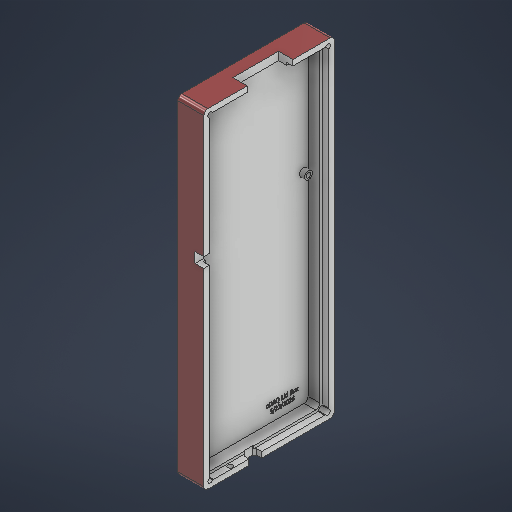
# Autodesk Inventor part: cDAQ_Lid_Box
Saved by Autodesk Inventor 2027 (Build 310192000, 192)
## iProperties
Created: 2026-05-08
Part Number: cDAQ_Lid_Box
Material: Generic
Document SubType Name: Modeling
Designer: giese
Density: 1 g/cm^3
Appearance: Default
Author: giese
Autodesk Inventor part; units mm, degrees
(part 1 of 2)
ref_plane "YZ Plane" through (0, 0, 0) normal (1, 0, 0) x (0, 1, 0)
ref_plane "XZ Plane" through (0, 0, 0) normal (0, 1, 0) x (-1, 0, 0)
ref_plane "XY Plane" through (0, 0, 0) normal (0, 0, 1) x (1, 0, 0)
sketch "Sketch1" plane through (0, 0, 0) normal (1, 0, 0) x (0, 1, 0)
  line L0 (50.7569, 48.4212) -> (-205.7831, 48.4212)
  line L1 (-205.7831, 48.4212) -> (-205.7831, -53.1788)
  line L2 (-205.7831, -53.1788) -> (50.7569, -53.1788)
  line L3 (50.7569, -53.1788) -> (50.7569, 48.4212)
  point P0 (0, 0)
  dimension "d0" = 101.6
  dimension "d1" = 256.54
  constraints: 8 end point, 2 parallel, 1 horizontal, 1 perpendicular
  measures "d0" distance of L2.end L0.start
  measures "d1" distance of L0.start L0.end
extrude "Extrusion1" add sketch "Sketch1" along normal blind 20.32
sketch "Sketch2" plane through (20.32, 0, 0) normal (1, 0, 0) x (0, 0, -1)
  line L0 (-42.0712, 44.4069) -> (46.8288, 44.4069)
  line L1 (46.8288, 44.4069) -> (46.8288, -199.4331)
  line L2 (46.8288, -199.4331) -> (-42.0712, -199.4331)
  line L3 (-42.0712, -199.4331) -> (-42.0712, 44.4069)
  line L4 (-48.4212, 50.7569) -> (-48.4212, -205.7831) projected
  line L5 (-48.4212, -205.7831) -> (53.1788, -205.7831) projected
  point P0 (0, 0)
  dimension "d4" = 88.9
  dimension "d5" = 243.84
  dimension "d6" = 6.35
  dimension "d7" = 6.35
  constraints: 8 end point, 2 parallel, 1 horizontal, 1 perpendicular
  measures "d4" distance of L0.start L0.end
  measures "d5" distance of L0.end L1.end
  measures "d6" distance between parallel lines of L4 L3
  measures "d7" distance between parallel lines of L5 L2
extrude "Extrusion2" cut sketch "Sketch2" against normal blind 13.97
sketch "Sketch3" plane through (0, 0, 0) normal (-1, 0, 0) x (0, 0, 1)
  circle A0 centre (-30.3188, 7.3229) radius 2
  line L0 (-53.1788, -205.7831) -> (-53.1788, 50.7569) projected
  line L1 (-53.1788, 50.7569) -> (48.4212, 50.7569) projected
  circle A1 centre (-11.82, 7.3229) radius 2
  circle A2 centre (6.6789, 7.3229) radius 2
  point P0 (0, 0)
  dimension "d10" = 22.86
  dimension "d11" = 43.434
  dimension "d12" = 43.434
  dimension "d13" = 18.4988
  dimension "d14" = 4
  dimension "d15" = 4
  dimension "d16" = 43.434
  dimension "d17" = 18.4988
  dimension "d18" = 36.9976
  dimension "d21" = 4
  constraints: 3 centre point
  measures "d10" distance from line of L0 A0.centre
  measures "d11" distance from line of L1 A0.centre
  measures "d12" distance from line of L1 A1.centre
  measures "d13" distance of A0.centre A1.centre
  measures "d14" diameter of A1
  measures "d15" diameter of A2
  measures "d16" distance from line of L1 A2.centre
  measures "d17" distance of A1.centre A2.centre
  measures "d18" distance of A0.centre A2.centre
  measures "d21" diameter of A0
extrude "Extrusion3" [suppressed]
sketch "Sketch6" plane through (0, 50.7569, 48.4212) normal (0, 1, 0) x (1, 0, 0)
  line L0 (20.32, 6.35) -> (20.32, 95.25) projected
  line L1 (9.144, 33.7719) -> (20.32, 33.7719)
  line L2 (20.32, 33.7719) -> (20.32, 69.342)
  line L3 (20.32, 69.342) -> (9.144, 69.342)
  line L4 (9.144, 69.342) -> (9.144, 33.7719)
  line L5 (0, 101.6) -> (20.32, 101.6) projected
  point P0 (0, 48.4212)
  point P1 (14.732, 69.342)
  point P2 (14.732, 33.7719)
  dimension "d30" = 11.176
  dimension "d31" = 35.5701
  dimension "d32" = 32.258
  constraints: 8 end point, 2 midpoint, 2 parallel, 1 horizontal, 1 perpendicular, 1 point on line
  measures "d30" distance between parallel lines of L0 L4
  measures "d31" distance of point (14.732, 69.342) point (14.732, 33.772)
  measures "d32" distance between parallel lines of L5 L3
extrude "Extrusion5" cut sketch "Sketch6" against normal blind 6.35
fillet "Fillet1" radius 3.175 4 edges at (10.16, 50.7569, -53.1788) (10.16, 50.7569, 48.4212) (10.16, -205.7831, 48.4212) (10.16, -205.7831, -53.1788)
sketch "Sketch7" plane through (20.32, 0, 0) normal (1, 0, 0) x (0, 0, -1)
  line L0 (-42.0712, -199.4331) -> (-42.0712, 44.4069) projected
  line L1 (-42.0712, 44.4069) -> (-42.3252, 44.4069)
  line L2 (-42.3252, 46.4069) -> (-44.0712, 46.4069)
  line L3 (-44.0712, 46.4069) -> (-44.0712, 51.0109)
  line L4 (-42.0712, -190.1621) -> (-42.0712, -199.4331)
  line L5 (46.8288, -199.4331) -> (-42.0712, -199.4331) projected
  line L6 (-40.4202, -201.4331) -> (-44.0712, -201.4331)
  line L7 (-44.0712, -201.4331) -> (-44.0712, -190.1621)
  line L8 (46.8288, 44.4069) -> (46.8288, -199.4331) projected
  line L9 (46.8288, -192.7021) -> (46.8288, -199.4331)
  line L10 (46.8288, -199.4331) -> (43.9078, -199.4331)
  line L11 (46.8288, -199.4331) -> (46.8288, -192.7021)
  line L12 (48.8288, -192.7021) -> (48.8288, -201.4331)
  line L13 (48.8288, -201.4331) -> (43.9078, -201.4331)
  line L14 (-42.0712, 44.4069) -> (46.8288, 44.4069) projected
  line L15 (42.0028, 44.4069) -> (46.8288, 44.4069)
  line L16 (48.8288, 48.4709) -> (48.8288, 46.4069)
  line L17 (48.8288, 46.4069) -> (42.0028, 46.4069)
  line L18 (-42.3252, 46.4069) -> (42.0028, 46.4069)
  line L19 (42.0028, 44.4069) -> (-42.3252, 44.4069)
  line L20 (48.8288, 48.4709) -> (48.8288, -192.7021)
  line L21 (44.2888, -195.2421) -> (44.2888, 44.4069)
  line L22 (43.9078, -199.4331) -> (-40.4202, -199.4331)
  line L23 (-40.4202, -201.4331) -> (43.9078, -201.4331)
  line L24 (-44.0712, -190.1621) -> (-44.0712, 51.0109)
  line L25 (-42.0712, 44.4069) -> (-42.0712, -190.1621)
  point P0 (0, 0)
  point P1 (-42.0712, 51.0109)
  point P2 (-44.2302, 48.9789)
  point P3 (46.8288, 48.4709)
  point P4 (48.8288, 46.4069)
  dimension "d34" = 2
  dimension "d35" = 2
  dimension "d38" = 2
  dimension "d39" = 2
  dimension "d42" = 2
  dimension "d43" = 2
  dimension "d46" = 2
  dimension "d47" = 2
  constraints: 44 end point, 9 point on line, 4 parallel, 4 perpendicular, 2 collinear, 2 horizontal, 2 vertical
  measures "d34" distance between parallel lines of L2 L1
  measures "d35" distance between parallel lines of L0 L3
  measures "d38" distance between parallel lines of L7 L0
  measures "d39" distance between parallel lines of L5 L6
  measures "d42" distance between parallel lines of L5 L13
  measures "d43" distance between parallel lines of L8 L12
  measures "d46" distance between parallel lines of L14 L17
  measures "d47" distance between parallel lines of L8 L16
extrude "Extrusion6" cut sketch "Sketch7" against normal blind 5 contours L0 L14 L8 L5 | L18 L17 L20 L12 L13 L23 L6 L7 L24 L2
fillet "Fillet2" radius 3.175 6 edges at (10.835, 44.4069, 42.0712) (10.835, 44.4069, -46.8288) (10.835, -199.4331, 42.0712) (17.82, -201.4331, 44.0712) (10.835, -199.4331, -46.8288) (17.82, -201.4331, -48.8288)
sketch "Sketch11" plane through (15.32, 0, 0) normal (1, 0, 0) x (0, 0, -1)
  circle A0 centre (48.0988, 45.6769) radius 1.9939
  line L0 (50.0038, 50.7569) -> (20.9208, 50.7569) projected
  line L1 (53.1788, -202.6081) -> (53.1788, 47.5819) projected
  arc A1 (46.9238, 45.7719) -> (43.7488, 48.9469) centre (43.7488, 45.7719) ccw projected
  circle A2 centre (-43.3412, 45.6769) radius 1.9939
  line L2 (-48.4212, 47.5819) -> (-48.4212, -202.6081) projected
  line L3 (-14.6493, 50.7569) -> (-45.2462, 50.7569) projected
  circle A3 centre (48.0988, -200.7031) radius 1.9939
  line L4 (-45.2462, -205.7831) -> (50.0038, -205.7831) projected
  circle A4 centre (-43.3412, -200.7031) radius 1.9939
  circle A5 centre (43.0188, -43.2231) radius 1.9939
  circle A6 centre (-38.2612, -43.2231) radius 1.9939
  point P0 (0, 0)
  point P1 (45.9939, 48.017)
  point P2 (48.5528, -43.2993)
  point P3 (45.3778, -46.4743)
  point P4 (-30.4007, -42.8803)
  point P5 (-33.5757, -46.0553)
  dimension "d58" = 3.9878
  dimension "d59" = 5.08
  dimension "d60" = 5.08
  dimension "d61" = 3.9878
  dimension "d62" = 3.9878
  dimension "d63" = 5.08
  dimension "d64" = 5.08
  dimension "d65" = 3.9878
  dimension "d66" = 5.08
  dimension "d67" = 5.08
  dimension "d76" = 5.08
  dimension "d77" = 5.08
  dimension "d114" = 3.9878
  dimension "d115" = 93.98
  dimension "d116" = 10.16
  dimension "d117" = 3.9878
  dimension "d118" = 93.98
  dimension "d119" = 10.16
  constraints: 6 centre point, 1 point on circle
  measures "d58" diameter of A0
  measures "d59" distance from line of L2 A2.centre
  measures "d60" distance from line of L3 A2.centre
  measures "d61" diameter of A2
  measures "d62" diameter of A3
  measures "d63" distance from line of L1 A3.centre
  measures "d64" distance from line of L4 A3.centre
  measures "d65" diameter of A4
  measures "d66" distance from line of L2 A4.centre
  measures "d67" distance from line of L4 A4.centre
  measures "d76" distance from line of L1 A0.centre
  measures "d77" distance from line of L0 A0.centre
  measures "d114" diameter of A5
  measures "d115" distance from line of A5.centre L0
  measures "d116" distance from line of L1 A5.centre
  measures "d117" diameter of A6
  measures "d118" distance from line of A6.centre L3
  measures "d119" distance from line of L2 A6.centre
extrude "Extrusion8" cut sketch "Sketch11" along normal blind 5.08 and the other way blind 17.78
sketch "Sketch13" plane through (6.35, 0, 0) normal (1, 0, 0) x (0, 0, -1)
  line L0 (14.1785, -185.2739) -> (39.2344, -185.2739) construction
  line L1 (39.2344, -185.2739) -> (39.2344, -194.1382) construction
  line L2 (39.2344, -194.1382) -> (14.1785, -194.1382) construction
  line L3 (14.1785, -194.1382) -> (14.1785, -185.2739) construction
  spline S0 degree 2 poles (15.3666, -188.5097) (15.1295, -188.5097) (14.7367, -188.3639) (14.5959, -188.2157) knots 0 0 0 1 2 2 2
  spline S1 degree 2 poles (14.5959, -188.2157) (14.4552, -188.07) (14.2995, -187.6205) (14.2995, -187.3191) knots 0 0 0 1 2 2 2
  spline S2 degree 2 poles (14.2995, -187.3191) (14.2995, -187.0178) (14.4601, -186.5781) (14.5959, -186.4299) knots 0 0 0 1 2 2 2
  spline S3 degree 2 poles (14.5959, -186.4299) (14.7318, -186.2792) (15.1344, -186.1187) (15.3666, -186.1187) knots 0 0 0 1 2 2 2
  spline S4 degree 2 poles (15.3666, -186.1187) (15.5543, -186.1187) (15.9051, -186.2249) (16.0409, -186.2941) knots 0 0 0 1 2 2 2
  line L4 (16.0409, -186.2941) -> (16.0409, -186.7263)
  line L5 (16.0409, -186.7263) -> (16.0187, -186.7263)
  spline S5 degree 2 poles (16.0187, -186.7263) (15.9767, -186.6917) (15.8482, -186.6028) (15.7569, -186.5559) knots 0 0 0 1 2 2 2
  spline S6 degree 2 poles (15.7569, -186.5559) (15.6753, -186.5164) (15.458, -186.4546) (15.3592, -186.4546) knots 0 0 0 1 2 2 2
  spline S7 degree 2 poles (15.3592, -186.4546) (15.0603, -186.4546) (14.6972, -186.9066) (14.6972, -187.3191) knots 0 0 0 1 2 2 2
  spline S8 degree 2 poles (14.6972, -187.3191) (14.6972, -187.7217) (15.048, -188.1737) (15.3592, -188.1737) knots 0 0 0 1 2 2 2
  spline S9 degree 2 poles (15.3592, -188.1737) (15.5469, -188.1737) (15.8878, -188.0181) (16.0187, -187.8971) knots 0 0 0 1 2 2 2
  line L6 (16.0187, -187.8971) -> (16.0409, -187.8971)
  line L7 (16.0409, -187.8971) -> (16.0409, -188.3293)
  spline S10 degree 2 poles (16.0409, -188.3293) (15.9841, -188.3565) (15.8112, -188.4331) (15.742, -188.4504) knots 0 0 0 1 2 2 2
  spline S11 degree 2 poles (15.742, -188.4504) (15.6432, -188.48) (15.4876, -188.5097) (15.3666, -188.5097) knots 0 0 0 1 2 2 2
  spline S12 degree 2 poles (18.8246, -186.9363) (18.8246, -187.3537) (18.4862, -188.0255) (18.2022, -188.2133) knots 0 0 0 1 2 2 2
  spline S13 degree 2 poles (18.2022, -188.2133) (17.97, -188.359) (17.4933, -188.4578) (17.1228, -188.4578) knots 0 0 0 1 2 2 2
  line L8 (17.1228, -188.4578) -> (16.4213, -188.4578)
  line L9 (16.4213, -188.4578) -> (16.4213, -185.4098)
  line L10 (16.4213, -185.4098) -> (17.1154, -185.4098)
  spline S14 degree 2 poles (17.1154, -185.4098) (17.5451, -185.4098) (18.0342, -185.5382) (18.2071, -185.6519) knots 0 0 0 1 2 2 2
  spline S15 degree 2 poles (18.2071, -185.6519) (18.501, -185.847) (18.8246, -186.4917) (18.8246, -186.9363) knots 0 0 0 1 2 2 2
  spline S16 degree 2 poles (18.4022, -186.9313) (18.4022, -186.5806) (18.1701, -186.0841) (17.9404, -185.9433) knots 0 0 0 1 2 2 2
  spline S17 degree 2 poles (17.9404, -185.9433) (17.7773, -185.847) (17.4093, -185.7605) (17.1351, -185.7605) knots 0 0 0 1 2 2 2
  line L11 (17.1351, -185.7605) -> (16.8264, -185.7605)
  line L12 (16.8264, -185.7605) -> (16.8264, -188.107)
  line L13 (16.8264, -188.107) -> (17.1351, -188.107)
  spline S18 degree 2 poles (17.1351, -188.107) (17.4044, -188.107) (17.8119, -188.0206) (17.9774, -187.9045) knots 0 0 0 1 2 2 2
  spline S19 degree 2 poles (17.9774, -187.9045) (18.1898, -187.7612) (18.4022, -187.287) (18.4022, -186.9313) knots 0 0 0 1 2 2 2
  line L14 (18.9358, -188.4578) -> (19.9633, -185.4098)
  line L15 (19.9633, -185.4098) -> (20.4622, -185.4098)
  line L16 (20.4622, -185.4098) -> (21.4898, -188.4578)
  line L17 (21.4898, -188.4578) -> (21.0625, -188.4578)
  line L18 (21.0625, -188.4578) -> (20.7858, -187.6056)
  line L19 (20.7858, -187.6056) -> (19.6224, -187.6056)
  line L20 (19.6224, -187.6056) -> (19.3458, -188.4578)
  line L21 (19.3458, -188.4578) -> (18.9358, -188.4578)
  line L22 (20.6747, -187.2598) -> (20.2029, -185.8248)
  line L23 (20.2029, -185.8248) -> (19.7336, -187.2598)
  line L24 (19.7336, -187.2598) -> (20.6747, -187.2598)
  spline S20 degree 2 poles (24.3105, -189.2037) (24.1994, -189.2309) (23.9573, -189.2605) (23.8363, -189.2605) knots 0 0 0 1 2 2 2
  spline S21 degree 2 poles (23.8363, -189.2605) (23.4929, -189.2605) (23.0656, -188.8777) (23.0459, -188.522) knots 0 0 0 1 2 2 2
  spline S22 degree 2 poles (23.0459, -188.522) (23.0187, -188.522) (22.9718, -188.522) (22.952, -188.522) knots 0 0 0 1 2 2 2
  spline S23 degree 2 poles (22.952, -188.522) (22.6433, -188.522) (22.1468, -188.3121) (21.9689, -188.107) knots 0 0 0 1 2 2 2
  spline S24 degree 2 poles (21.9689, -188.107) (21.7936, -187.9045) (21.6059, -187.3117) (21.6059, -186.9363) knots 0 0 0 1 2 2 2
  spline S25 degree 2 poles (21.6059, -186.9363) (21.6059, -186.5509) (21.796, -185.968) (21.9714, -185.7605) knots 0 0 0 1 2 2 2
  spline S26 degree 2 poles (21.9714, -185.7605) (22.1493, -185.5555) (22.6457, -185.3456) (22.952, -185.3456) knots 0 0 0 1 2 2 2
  spline S27 degree 2 poles (22.952, -185.3456) (23.2632, -185.3456) (23.7622, -185.5629) (23.9351, -185.7605) knots 0 0 0 1 2 2 2
  spline S28 degree 2 poles (23.9351, -185.7605) (24.108, -185.9606) (24.3006, -186.5559) (24.3006, -186.9363) knots 0 0 0 1 2 2 2
  spline S29 degree 2 poles (24.3006, -186.9363) (24.3006, -187.5291) (23.8387, -188.2997) (23.4361, -188.4356) knots 0 0 0 1 2 2 2
  spline S30 degree 2 poles (23.4361, -188.4356) (23.446, -188.5492) (23.5053, -188.732) (23.5522, -188.7838) knots 0 0 0 1 2 2 2
  spline S31 degree 2 poles (23.5522, -188.7838) (23.609, -188.8481) (23.7646, -188.9073) (23.903, -188.9073) knots 0 0 0 1 2 2 2
  spline S32 degree 2 poles (23.903, -188.9073) (23.9845, -188.9073) (24.2068, -188.8555) (24.2562, -188.8357) knots 0 0 0 1 2 2 2
  line L25 (24.2562, -188.8357) -> (24.3105, -188.8357)
  line L26 (24.3105, -188.8357) -> (24.3105, -189.2037)
  spline S33 degree 2 poles (23.8783, -186.9363) (23.8783, -186.6324) (23.7474, -186.1656) (23.6288, -186.0125) knots 0 0 0 1 2 2 2
  spline S34 degree 2 poles (23.6288, -186.0125) (23.5078, -185.8544) (23.1669, -185.6963) (22.9545, -185.6963) knots 0 0 0 1 2 2 2
  spline S35 degree 2 poles (22.9545, -185.6963) (22.7347, -185.6963) (22.4037, -185.8495) (22.2777, -186.0125) knots 0 0 0 1 2 2 2
  spline S36 degree 2 poles (22.2777, -186.0125) (22.1567, -186.1681) (22.0282, -186.6399) (22.0282, -186.9363) knots 0 0 0 1 2 2 2
  spline S37 degree 2 poles (22.0282, -186.9363) (22.0282, -187.5365) (22.5321, -188.1762) (22.9545, -188.1762) knots 0 0 0 1 2 2 2
  spline S38 degree 2 poles (22.9545, -188.1762) (23.3769, -188.1762) (23.8783, -187.5365) (23.8783, -186.9363) knots 0 0 0 1 2 2 2
  line L27 (27.8204, -188.4578) -> (26.0544, -188.4578)
  line L28 (26.0544, -188.4578) -> (26.0544, -185.4098)
  line L29 (26.0544, -185.4098) -> (26.4594, -185.4098)
  line L30 (26.4594, -185.4098) -> (26.4594, -188.0972)
  line L31 (26.4594, -188.0972) -> (27.8204, -188.0972)
  line L32 (27.8204, -188.0972) -> (27.8204, -188.4578)
  line L33 (28.5021, -188.4578) -> (28.1168, -188.4578)
  line L34 (28.1168, -188.4578) -> (28.1168, -186.1706)
  line L35 (28.1168, -186.1706) -> (28.5021, -186.1706)
  line L36 (28.5021, -186.1706) -> (28.5021, -188.4578)
  line L37 (28.5293, -185.7902) -> (28.0921, -185.7902)
  line L38 (28.0921, -185.7902) -> (28.0921, -185.39)
  line L39 (28.0921, -185.39) -> (28.5293, -185.39)
  line L40 (28.5293, -185.39) -> (28.5293, -185.7902)
  line L41 (30.8264, -188.4578) -> (30.4411, -188.4578)
  line L42 (30.4411, -188.4578) -> (30.4411, -188.2256)
  spline S39 degree 2 poles (30.4411, -188.2256) (30.3522, -188.2997) (30.2213, -188.3985) (30.1324, -188.4405) knots 0 0 0 1 2 2 2
  spline S40 degree 2 poles (30.1324, -188.4405) (30.0508, -188.48) (29.8755, -188.522) (29.7594, -188.522) knots 0 0 0 1 2 2 2
  spline S41 degree 2 poles (29.7594, -188.522) (29.5717, -188.522) (29.2555, -188.3664) (29.1443, -188.2157) knots 0 0 0 1 2 2 2
  spline S42 degree 2 poles (29.1443, -188.2157) (29.0332, -188.0651) (28.9097, -187.6205) (28.9097, -187.3315) knots 0 0 0 1 2 2 2
  spline S43 degree 2 poles (28.9097, -187.3315) (28.9097, -187.0301) (29.0653, -186.5905) (29.2012, -186.425) knots 0 0 0 1 2 2 2
  spline S44 degree 2 poles (29.2012, -186.425) (29.3271, -186.2768) (29.6803, -186.1063) (29.8755, -186.1063) knots 0 0 0 1 2 2 2
  spline S45 degree 2 poles (29.8755, -186.1063) (30.0459, -186.1063) (30.3003, -186.1829) (30.4411, -186.2619) knots 0 0 0 1 2 2 2
  line L43 (30.4411, -186.2619) -> (30.4411, -185.2739)
  line L44 (30.4411, -185.2739) -> (30.8264, -185.2739)
  line L45 (30.8264, -185.2739) -> (30.8264, -188.4578)
  line L46 (30.4411, -187.902) -> (30.4411, -186.5806)
  spline S46 degree 2 poles (30.4411, -186.5806) (30.2978, -186.5114) (30.0706, -186.4595) (29.9397, -186.4595) knots 0 0 0 1 2 2 2
  spline S47 degree 2 poles (29.9397, -186.4595) (29.6433, -186.4595) (29.3074, -186.9041) (29.3074, -187.3241) knots 0 0 0 1 2 2 2
  spline S48 degree 2 poles (29.3074, -187.3241) (29.3074, -187.7291) (29.5642, -188.1564) (29.8483, -188.1564) knots 0 0 0 1 2 2 2
  spline S49 degree 2 poles (29.8483, -188.1564) (29.999, -188.1564) (30.3053, -188.0181) (30.4411, -187.902) knots 0 0 0 1 2 2 2
  spline S50 degree 2 poles (34.7908, -187.5217) (34.7908, -187.7489) (34.6179, -188.0972) (34.4746, -188.2108) knots 0 0 0 1 2 2 2
  spline S51 degree 2 poles (34.4746, -188.2108) (34.3017, -188.3442) (33.909, -188.4578) (33.5978, -188.4578) knots 0 0 0 1 2 2 2
  line L47 (33.5978, -188.4578) -> (32.7234, -188.4578)
  line L48 (32.7234, -188.4578) -> (32.7234, -185.4098)
  line L49 (32.7234, -185.4098) -> (33.5311, -185.4098)
  spline S52 degree 2 poles (33.5311, -185.4098) (33.8571, -185.4098) (34.1832, -185.4518) (34.3314, -185.5333) knots 0 0 0 1 2 2 2
  spline S53 degree 2 poles (34.3314, -185.5333) (34.4969, -185.6197) (34.6475, -185.9038) (34.6475, -186.0965) knots 0 0 0 1 2 2 2
  spline S54 degree 2 poles (34.6475, -186.0965) (34.6475, -186.3113) (34.4203, -186.6522) (34.2202, -186.7485) knots 0 0 0 1 2 2 2
  line L50 (34.2202, -186.7485) -> (34.2202, -186.7634)
  spline S55 degree 2 poles (34.2202, -186.7634) (34.4919, -186.8375) (34.7908, -187.2302) (34.7908, -187.5217) knots 0 0 0 1 2 2 2
  spline S56 degree 2 poles (34.3684, -187.5389) (34.3684, -187.366) (34.2696, -187.1437) (34.1214, -187.0647) knots 0 0 0 1 2 2 2
  spline S57 degree 2 poles (34.1214, -187.0647) (34.0251, -187.0153) (33.7979, -186.9857) (33.5879, -186.9857) knots 0 0 0 1 2 2 2
  line L51 (33.5879, -186.9857) -> (33.1285, -186.9857)
  line L52 (33.1285, -186.9857) -> (33.1285, -188.112)
  line L53 (33.1285, -188.112) -> (33.457, -188.112)
  spline S58 degree 2 poles (33.457, -188.112) (33.7238, -188.112) (34.03, -188.0626) (34.1486, -187.9835) knots 0 0 0 1 2 2 2
  spline S59 degree 2 poles (34.1486, -187.9835) (34.2622, -187.902) (34.3684, -187.6995) (34.3684, -187.5389) knots 0 0 0 1 2 2 2
  spline S60 degree 2 poles (34.2252, -186.1533) (34.2252, -186.0446) (34.1511, -185.8816) (34.0696, -185.8346) knots 0 0 0 1 2 2 2
  spline S61 degree 2 poles (34.0696, -185.8346) (33.9708, -185.7803) (33.7312, -185.7556) (33.5163, -185.7556) knots 0 0 0 1 2 2 2
  line L54 (33.5163, -185.7556) -> (33.1285, -185.7556)
  line L55 (33.1285, -185.7556) -> (33.1285, -186.6473)
  line L56 (33.1285, -186.6473) -> (33.5879, -186.6473)
  spline S62 degree 2 poles (33.5879, -186.6473) (33.7781, -186.6473) (33.9584, -186.6077) (34.0547, -186.546) knots 0 0 0 1 2 2 2
  spline S63 degree 2 poles (34.0547, -186.546) (34.1486, -186.4867) (34.2252, -186.2965) (34.2252, -186.1533) knots 0 0 0 1 2 2 2
  spline S64 degree 2 poles (37.0435, -187.3142) (37.0435, -187.8922) (36.4877, -188.522) (36.0233, -188.522) knots 0 0 0 1 2 2 2
  spline S65 degree 2 poles (36.0233, -188.522) (35.5466, -188.522) (35.0008, -187.8724) (35.0008, -187.3142) knots 0 0 0 1 2 2 2
  spline S66 degree 2 poles (35.0008, -187.3142) (35.0008, -186.7411) (35.5639, -186.1063) (36.0233, -186.1063) knots 0 0 0 1 2 2 2
  spline S67 degree 2 poles (36.0233, -186.1063) (36.4877, -186.1063) (37.0435, -186.7387) (37.0435, -187.3142) knots 0 0 0 1 2 2 2
  spline S68 degree 2 poles (36.6458, -187.3142) (36.6458, -186.8696) (36.3222, -186.4373) (36.0233, -186.4373) knots 0 0 0 1 2 2 2
  spline S69 degree 2 poles (36.0233, -186.4373) (35.7245, -186.4373) (35.3984, -186.8696) (35.3984, -187.3142) knots 0 0 0 1 2 2 2
  spline S70 degree 2 poles (35.3984, -187.3142) (35.3984, -187.7464) (35.7245, -188.191) (36.0233, -188.191) knots 0 0 0 1 2 2 2
  spline S71 degree 2 poles (36.0233, -188.191) (36.3197, -188.191) (36.6458, -187.7538) (36.6458, -187.3142) knots 0 0 0 1 2 2 2
  line L57 (39.2146, -188.4578) -> (38.7428, -188.4578)
  line L58 (38.7428, -188.4578) -> (38.1871, -187.5982)
  line L59 (38.1871, -187.5982) -> (37.6165, -188.4578)
  line L60 (37.6165, -188.4578) -> (37.1793, -188.4578)
  line L61 (37.1793, -188.4578) -> (37.9722, -187.3241)
  line L62 (37.9722, -187.3241) -> (37.1867, -186.1706)
  line L63 (37.1867, -186.1706) -> (37.6585, -186.1706)
  line L64 (37.6585, -186.1706) -> (38.2118, -187.0227)
  line L65 (38.2118, -187.0227) -> (38.7774, -186.1706)
  line L66 (38.7774, -186.1706) -> (39.2146, -186.1706)
  line L67 (39.2146, -186.1706) -> (38.4267, -187.2994)
  line L68 (38.4267, -187.2994) -> (39.2146, -188.4578)
  spline S72 degree 2 poles (19.1679, -192.508) (19.1679, -192.7278) (19.0272, -193.1033) (18.8987, -193.2416) knots 0 0 0 1 2 2 2
  spline S73 degree 2 poles (18.8987, -193.2416) (18.7703, -193.3799) (18.3874, -193.5405) (18.1503, -193.5405) knots 0 0 0 1 2 2 2
  spline S74 degree 2 poles (18.1503, -193.5405) (17.9329, -193.5405) (17.5081, -193.4441) (17.3525, -193.3676) knots 0 0 0 1 2 2 2
  line L69 (17.3525, -193.3676) -> (17.3525, -192.9353)
  line L70 (17.3525, -192.9353) -> (17.3821, -192.9353)
  spline S75 degree 2 poles (17.3821, -192.9353) (17.4291, -192.9699) (17.6044, -193.0588) (17.7106, -193.0983) knots 0 0 0 1 2 2 2
  spline S76 degree 2 poles (17.7106, -193.0983) (17.8317, -193.1403) (18.0317, -193.1872) (18.1577, -193.1872) knots 0 0 0 1 2 2 2
  spline S77 degree 2 poles (18.1577, -193.1872) (18.2812, -193.1872) (18.5134, -193.0983) (18.5974, -193.002) knots 0 0 0 1 2 2 2
  spline S78 degree 2 poles (18.5974, -193.002) (18.6739, -192.9106) (18.753, -192.6685) (18.753, -192.5055) knots 0 0 0 1 2 2 2
  spline S79 degree 2 poles (18.753, -192.5055) (18.753, -192.3425) (18.6641, -192.135) (18.5801, -192.0659) knots 0 0 0 1 2 2 2
  spline S80 degree 2 poles (18.5801, -192.0659) (18.4936, -191.9893) (18.2368, -191.9251) (18.0811, -191.9251) knots 0 0 0 1 2 2 2
  spline S81 degree 2 poles (18.0811, -191.9251) (17.9132, -191.9251) (17.5797, -191.9769) (17.4785, -191.9992) knots 0 0 0 1 2 2 2
  line L71 (17.4785, -191.9992) -> (17.4785, -190.4282)
  line L72 (17.4785, -190.4282) -> (19.1507, -190.4282)
  line L73 (19.1507, -190.4282) -> (19.1507, -190.7864)
  line L74 (19.1507, -190.7864) -> (17.8712, -190.7864)
  line L75 (17.8712, -190.7864) -> (17.8712, -191.599)
  spline S82 degree 2 poles (17.8712, -191.599) (17.9453, -191.5891) (18.0886, -191.5817) (18.1478, -191.5817) knots 0 0 0 1 2 2 2
  spline S83 degree 2 poles (18.1478, -191.5817) (18.3825, -191.5817) (18.7061, -191.6583) (18.8543, -191.7719) knots 0 0 0 1 2 2 2
  spline S84 degree 2 poles (18.8543, -191.7719) (19.0049, -191.8856) (19.1679, -192.2314) (19.1679, -192.508) knots 0 0 0 1 2 2 2
  line L76 (20.8747, -190.2924) -> (19.6817, -194.1382)
  line L77 (19.6817, -194.1382) -> (19.3359, -194.1382)
  line L78 (19.3359, -194.1382) -> (20.524, -190.2924)
  line L79 (20.524, -190.2924) -> (20.8747, -190.2924)
  line L80 (23.0903, -193.4762) -> (21.2107, -193.4762)
  line L81 (21.2107, -193.4762) -> (21.2107, -193.044)
  spline S85 degree 2 poles (21.2107, -193.044) (21.4132, -192.8538) (21.7738, -192.5006) (21.9467, -192.3104) knots 0 0 0 1 2 2 2
  spline S86 degree 2 poles (21.9467, -192.3104) (22.295, -191.9275) (22.5494, -191.4681) (22.5494, -191.2236) knots 0 0 0 1 2 2 2
  spline S87 degree 2 poles (22.5494, -191.2236) (22.5494, -191.0951) (22.4704, -190.9025) (22.3987, -190.8407) knots 0 0 0 1 2 2 2
  spline S88 degree 2 poles (22.3987, -190.8407) (22.3271, -190.779) (22.1394, -190.7172) (22.0258, -190.7172) knots 0 0 0 1 2 2 2
  spline S89 degree 2 poles (22.0258, -190.7172) (21.9171, -190.7172) (21.6948, -190.7716) (21.5935, -190.8136) knots 0 0 0 1 2 2 2
  spline S90 degree 2 poles (21.5935, -190.8136) (21.5071, -190.8481) (21.3465, -190.9469) (21.2971, -190.9815) knots 0 0 0 1 2 2 2
  line L82 (21.2971, -190.9815) -> (21.2749, -190.9815)
  line L83 (21.2749, -190.9815) -> (21.2749, -190.5468)
  spline S91 degree 2 poles (21.2749, -190.5468) (21.4008, -190.4851) (21.8529, -190.364) (22.0554, -190.364) knots 0 0 0 1 2 2 2
  spline S92 degree 2 poles (22.0554, -190.364) (22.4827, -190.364) (22.9644, -190.816) (22.9644, -191.2014) knots 0 0 0 1 2 2 2
  spline S93 degree 2 poles (22.9644, -191.2014) (22.9644, -191.3817) (22.8804, -191.683) (22.8063, -191.8114) knots 0 0 0 1 2 2 2
  spline S94 degree 2 poles (22.8063, -191.8114) (22.7322, -191.9448) (22.5173, -192.2067) (22.3987, -192.3326) knots 0 0 0 1 2 2 2
  spline S95 degree 2 poles (22.3987, -192.3326) (22.2061, -192.5426) (21.7343, -192.9921) (21.5935, -193.123) knots 0 0 0 1 2 2 2
  line L84 (21.5935, -193.123) -> (23.0903, -193.123)
  line L85 (23.0903, -193.123) -> (23.0903, -193.4762)
  line L86 (25.3776, -193.4762) -> (23.4979, -193.4762)
  line L87 (23.4979, -193.4762) -> (23.4979, -193.044)
  spline S96 degree 2 poles (23.4979, -193.044) (23.7004, -192.8538) (24.0611, -192.5006) (24.234, -192.3104) knots 0 0 0 1 2 2 2
  spline S97 degree 2 poles (24.234, -192.3104) (24.5822, -191.9275) (24.8366, -191.4681) (24.8366, -191.2236) knots 0 0 0 1 2 2 2
  spline S98 degree 2 poles (24.8366, -191.2236) (24.8366, -191.0951) (24.7576, -190.9025) (24.686, -190.8407) knots 0 0 0 1 2 2 2
  spline S99 degree 2 poles (24.686, -190.8407) (24.6143, -190.779) (24.4266, -190.7172) (24.313, -190.7172) knots 0 0 0 1 2 2 2
  spline S100 degree 2 poles (24.313, -190.7172) (24.2043, -190.7172) (23.982, -190.7716) (23.8807, -190.8136) knots 0 0 0 1 2 2 2
  spline S101 degree 2 poles (23.8807, -190.8136) (23.7943, -190.8481) (23.6337, -190.9469) (23.5843, -190.9815) knots 0 0 0 1 2 2 2
  line L88 (23.5843, -190.9815) -> (23.5621, -190.9815)
  line L89 (23.5621, -190.9815) -> (23.5621, -190.5468)
  spline S102 degree 2 poles (23.5621, -190.5468) (23.6881, -190.4851) (24.1401, -190.364) (24.3426, -190.364) knots 0 0 0 1 2 2 2
  spline S103 degree 2 poles (24.3426, -190.364) (24.7699, -190.364) (25.2516, -190.816) (25.2516, -191.2014) knots 0 0 0 1 2 2 2
  spline S104 degree 2 poles (25.2516, -191.2014) (25.2516, -191.3817) (25.1676, -191.683) (25.0935, -191.8114) knots 0 0 0 1 2 2 2
  spline S105 degree 2 poles (25.0935, -191.8114) (25.0194, -191.9448) (24.8045, -192.2067) (24.686, -192.3326) knots 0 0 0 1 2 2 2
  spline S106 degree 2 poles (24.686, -192.3326) (24.4933, -192.5426) (24.0215, -192.9921) (23.8807, -193.123) knots 0 0 0 1 2 2 2
  line L90 (23.8807, -193.123) -> (25.3776, -193.123)
  line L91 (25.3776, -193.123) -> (25.3776, -193.4762)
  line L92 (27.0522, -190.2924) -> (25.8592, -194.1382)
  line L93 (25.8592, -194.1382) -> (25.5134, -194.1382)
  line L94 (25.5134, -194.1382) -> (26.7015, -190.2924)
  line L95 (26.7015, -190.2924) -> (27.0522, -190.2924)
  line L96 (29.2678, -193.4762) -> (27.3882, -193.4762)
  line L97 (27.3882, -193.4762) -> (27.3882, -193.044)
  spline S107 degree 2 poles (27.3882, -193.044) (27.5907, -192.8538) (27.9513, -192.5006) (28.1242, -192.3104) knots 0 0 0 1 2 2 2
  spline S108 degree 2 poles (28.1242, -192.3104) (28.4725, -191.9275) (28.7269, -191.4681) (28.7269, -191.2236) knots 0 0 0 1 2 2 2
  spline S109 degree 2 poles (28.7269, -191.2236) (28.7269, -191.0951) (28.6479, -190.9025) (28.5762, -190.8407) knots 0 0 0 1 2 2 2
  spline S110 degree 2 poles (28.5762, -190.8407) (28.5046, -190.779) (28.3169, -190.7172) (28.2033, -190.7172) knots 0 0 0 1 2 2 2
  spline S111 degree 2 poles (28.2033, -190.7172) (28.0946, -190.7172) (27.8723, -190.7716) (27.771, -190.8136) knots 0 0 0 1 2 2 2
  spline S112 degree 2 poles (27.771, -190.8136) (27.6846, -190.8481) (27.524, -190.9469) (27.4746, -190.9815) knots 0 0 0 1 2 2 2
  line L98 (27.4746, -190.9815) -> (27.4524, -190.9815)
  line L99 (27.4524, -190.9815) -> (27.4524, -190.5468)
  spline S113 degree 2 poles (27.4524, -190.5468) (27.5784, -190.4851) (28.0304, -190.364) (28.2329, -190.364) knots 0 0 0 1 2 2 2
  spline S114 degree 2 poles (28.2329, -190.364) (28.6602, -190.364) (29.1419, -190.816) (29.1419, -191.2014) knots 0 0 0 1 2 2 2
  spline S115 degree 2 poles (29.1419, -191.2014) (29.1419, -191.3817) (29.0579, -191.683) (28.9838, -191.8114) knots 0 0 0 1 2 2 2
  spline S116 degree 2 poles (28.9838, -191.8114) (28.9097, -191.9448) (28.6948, -192.2067) (28.5762, -192.3326) knots 0 0 0 1 2 2 2
  spline S117 degree 2 poles (28.5762, -192.3326) (28.3836, -192.5426) (27.9118, -192.9921) (27.771, -193.123) knots 0 0 0 1 2 2 2
  line L100 (27.771, -193.123) -> (29.2678, -193.123)
  line L101 (29.2678, -193.123) -> (29.2678, -193.4762)
  spline S118 degree 2 poles (31.5724, -191.9522) (31.5724, -192.7723) (31.0957, -193.5405) (30.5992, -193.5405) knots 0 0 0 1 2 2 2
  spline S119 degree 2 poles (30.5992, -193.5405) (30.0953, -193.5405) (29.6235, -192.7575) (29.6235, -191.9547) knots 0 0 0 1 2 2 2
  spline S120 degree 2 poles (29.6235, -191.9547) (29.6235, -191.1297) (30.1002, -190.3665) (30.5992, -190.3665) knots 0 0 0 1 2 2 2
  spline S121 degree 2 poles (30.5992, -190.3665) (31.1006, -190.3665) (31.5724, -191.1569) (31.5724, -191.9522) knots 0 0 0 1 2 2 2
  spline S122 degree 2 poles (31.0487, -192.881) (31.108, -192.7303) (31.1574, -192.2659) (31.1574, -191.9522) knots 0 0 0 1 2 2 2
  spline S123 degree 2 poles (31.1574, -191.9522) (31.1574, -191.6385) (31.108, -191.1767) (31.0463, -191.021) knots 0 0 0 1 2 2 2
  spline S124 degree 2 poles (31.0463, -191.021) (30.9845, -190.8654) (30.7696, -190.7049) (30.5992, -190.7049) knots 0 0 0 1 2 2 2
  spline S125 degree 2 poles (30.5992, -190.7049) (30.4288, -190.7049) (30.2089, -190.8654) (30.1447, -191.026) knots 0 0 0 1 2 2 2
  spline S126 degree 2 poles (30.1447, -191.026) (30.083, -191.1816) (30.0385, -191.6558) (30.0385, -191.9547) knots 0 0 0 1 2 2 2
  spline S127 degree 2 poles (30.0385, -191.9547) (30.0385, -192.2758) (30.078, -192.7056) (30.1422, -192.8736) knots 0 0 0 1 2 2 2
  spline S128 degree 2 poles (30.1422, -192.8736) (30.2015, -193.0316) (30.4213, -193.2021) (30.5992, -193.2021) knots 0 0 0 1 2 2 2
  spline S129 degree 2 poles (30.5992, -193.2021) (30.7671, -193.2021) (30.987, -193.0415) (31.0487, -192.881) knots 0 0 0 1 2 2 2
  line L102 (33.8423, -193.4762) -> (31.9626, -193.4762)
  line L103 (31.9626, -193.4762) -> (31.9626, -193.044)
  spline S130 degree 2 poles (31.9626, -193.044) (32.1652, -192.8538) (32.5258, -192.5006) (32.6987, -192.3104) knots 0 0 0 1 2 2 2
  spline S131 degree 2 poles (32.6987, -192.3104) (33.047, -191.9275) (33.3014, -191.4681) (33.3014, -191.2236) knots 0 0 0 1 2 2 2
  spline S132 degree 2 poles (33.3014, -191.2236) (33.3014, -191.0951) (33.2223, -190.9025) (33.1507, -190.8407) knots 0 0 0 1 2 2 2
  spline S133 degree 2 poles (33.1507, -190.8407) (33.0791, -190.779) (32.8914, -190.7172) (32.7777, -190.7172) knots 0 0 0 1 2 2 2
  spline S134 degree 2 poles (32.7777, -190.7172) (32.6691, -190.7172) (32.4468, -190.7716) (32.3455, -190.8136) knots 0 0 0 1 2 2 2
  spline S135 degree 2 poles (32.3455, -190.8136) (32.259, -190.8481) (32.0985, -190.9469) (32.0491, -190.9815) knots 0 0 0 1 2 2 2
  line L104 (32.0491, -190.9815) -> (32.0269, -190.9815)
  line L105 (32.0269, -190.9815) -> (32.0269, -190.5468)
  spline S136 degree 2 poles (32.0269, -190.5468) (32.1528, -190.4851) (32.6048, -190.364) (32.8074, -190.364) knots 0 0 0 1 2 2 2
  spline S137 degree 2 poles (32.8074, -190.364) (33.2347, -190.364) (33.7163, -190.816) (33.7163, -191.2014) knots 0 0 0 1 2 2 2
  spline S138 degree 2 poles (33.7163, -191.2014) (33.7163, -191.3817) (33.6324, -191.683) (33.5583, -191.8114) knots 0 0 0 1 2 2 2
  spline S139 degree 2 poles (33.5583, -191.8114) (33.4842, -191.9448) (33.2693, -192.2067) (33.1507, -192.3326) knots 0 0 0 1 2 2 2
  spline S140 degree 2 poles (33.1507, -192.3326) (32.958, -192.5426) (32.4863, -192.9921) (32.3455, -193.123) knots 0 0 0 1 2 2 2
  line L106 (32.3455, -193.123) -> (33.8423, -193.123)
  line L107 (33.8423, -193.123) -> (33.8423, -193.4762)
  spline S141 degree 2 poles (36.1765, -192.4882) (36.1765, -192.7229) (36.0209, -193.1206) (35.89, -193.2539) knots 0 0 0 1 2 2 2
  spline S142 degree 2 poles (35.89, -193.2539) (35.7541, -193.3947) (35.4132, -193.5405) (35.2082, -193.5405) knots 0 0 0 1 2 2 2
  spline S143 degree 2 poles (35.2082, -193.5405) (35.0032, -193.5405) (34.6648, -193.4021) (34.5364, -193.2638) knots 0 0 0 1 2 2 2
  spline S144 degree 2 poles (34.5364, -193.2638) (34.3783, -193.0983) (34.2005, -192.5426) (34.2005, -192.1375) knots 0 0 0 1 2 2 2
  spline S145 degree 2 poles (34.2005, -192.1375) (34.2005, -191.7398) (34.3635, -191.1001) (34.5339, -190.863) knots 0 0 0 1 2 2 2
  spline S146 degree 2 poles (34.5339, -190.863) (34.6994, -190.6308) (35.2231, -190.3714) (35.5664, -190.3714) knots 0 0 0 1 2 2 2
  spline S147 degree 2 poles (35.5664, -190.3714) (35.6677, -190.3714) (35.8455, -190.3912) (35.9122, -190.4134) knots 0 0 0 1 2 2 2
  line L108 (35.9122, -190.4134) -> (35.9122, -190.8062)
  line L109 (35.9122, -190.8062) -> (35.8949, -190.8062)
  spline S148 degree 2 poles (35.8949, -190.8062) (35.8381, -190.7765) (35.6306, -190.7246) (35.512, -190.7246) knots 0 0 0 1 2 2 2
  spline S149 degree 2 poles (35.512, -190.7246) (35.1317, -190.7246) (34.6648, -191.2384) (34.6204, -191.7423) knots 0 0 0 1 2 2 2
  spline S150 degree 2 poles (34.6204, -191.7423) (34.7661, -191.641) (35.0724, -191.5299) (35.2552, -191.5299) knots 0 0 0 1 2 2 2
  spline S151 degree 2 poles (35.2552, -191.5299) (35.433, -191.5299) (35.6998, -191.6015) (35.8455, -191.7102) knots 0 0 0 1 2 2 2
  spline S152 degree 2 poles (35.8455, -191.7102) (36.0135, -191.8362) (36.1765, -192.2264) (36.1765, -192.4882) knots 0 0 0 1 2 2 2
  spline S153 degree 2 poles (35.7615, -192.5055) (35.7615, -192.3178) (35.6627, -192.0634) (35.554, -191.9745) knots 0 0 0 1 2 2 2
  spline S154 degree 2 poles (35.554, -191.9745) (35.4725, -191.9103) (35.27, -191.8683) (35.1638, -191.8683) knots 0 0 0 1 2 2 2
  spline S155 degree 2 poles (35.1638, -191.8683) (35.0205, -191.8683) (34.7513, -191.9547) (34.6204, -192.0362) knots 0 0 0 1 2 2 2
  spline S156 degree 2 poles (34.6204, -192.0362) (34.6179, -192.0807) (34.613, -192.1647) (34.613, -192.2289) knots 0 0 0 1 2 2 2
  spline S157 degree 2 poles (34.613, -192.2289) (34.613, -192.545) (34.7365, -192.9328) (34.8303, -193.0341) knots 0 0 0 1 2 2 2
  spline S158 degree 2 poles (34.8303, -193.0341) (34.9168, -193.1304) (35.1045, -193.207) (35.2107, -193.207) knots 0 0 0 1 2 2 2
  spline S159 degree 2 poles (35.2107, -193.207) (35.4577, -193.207) (35.7615, -192.8563) (35.7615, -192.5055) knots 0 0 0 1 2 2 2
  point P0 (0, 0)
  constraints: 2 other
emboss "Emboss1" sketch "Sketch13" operation cut depth 2.54 direction (-1, 0, 0)